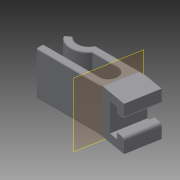
# Autodesk Inventor part: pinza
Saved by Autodesk Inventor 2015 SP1 (Build 190203100, 203)
## iProperties
Created: 2015-12-16
Part Number: pinza
Material: Generic
Document SubType Name: Modeling
Designer: pc
Density: 1 g/cm^3
Appearance: Default
Author: pc
Autodesk Inventor part; units mm, degrees
ref_plane "YZ Plane" through (0, 0, 0) normal (1, 0, 0) x (0, 1, 0)
ref_plane "XZ Plane" through (0, 0, 0) normal (0, 1, 0) x (-1, 0, 0)
ref_plane "XY Plane" through (0, 0, 0) normal (0, 0, 1) x (1, 0, 0)
sketch "Sketch1" plane through (0, 0, 0) normal (0, 0, 1) x (1, 0, 0)
  line L0 (-13.4572, -6) -> (9.0428, -6)
  line L1 (9.0428, -6) -> (9.0428, 0)
  line L2 (9.0428, 0) -> (-2.5, 0)
  arc A0 (-12.5, 0) -> (-2.5, 0) centre (-7.5, 3.75) ccw
  arc A1 (-10.5, 1.5) -> (-3.9645, 2.5) centre (-7.5, 3.75) ccw
  line L3 (-3.9645, 2.5) -> (11.5428, 2.5)
  line L4 (11.5428, 2.5) -> (11.5428, -8.5)
  line L5 (11.5428, -8.5) -> (-13.4572, -8.5)
  line L6 (-13.4572, -6) -> (-13.4572, -8.5)
  line L7 (-12.5, 0) -> (-10.5, 1.5)
  point P0 (0, 0)
  dimension "d4" = 6
  dimension "d5" = 25
  constraints: 16 end point, 4 point on circle, 2 centre point, 2 perpendicular, 1 horizontal, 1 vertical, 3 other
  measures "d4" distance of L0.end L1.end
  measures "d5" distance of L4.end L5.end
extrude "Extrusion1" add sketch "Sketch1" along normal blind 15
ref_plane "Work Plane1" through (11.5428, 2.5, 0) normal (0.9848078, -0.1736482, 0) x (0, 0, 1)
sketch "Sketch3" plane through (0, 0, 0) normal (0, 0, -1) x (-1, 0, 0)
  line L0 (-8.3381, -15.6747) -> (-12.3263, 6.9435) projected
  line L1 (13.4572, -6) -> (-9.0428, -6) projected
  line L2 (-9.0428, -6) -> (-9.0428, 0) projected
  line L3 (-9.0428, 0) -> (2.5, 0) projected
  arc A0 (2.5, 0) -> (12.5, 0) centre (7.5, 3.75) ccw projected
  line L4 (12.5, 0) -> (10.5, 1.5) projected
  arc A1 (3.9645, 2.5) -> (10.5, 1.5) centre (7.5, 3.75) ccw projected
  line L5 (3.9645, 2.5) -> (-11.5428, 2.5) projected
  line L6 (-11.5428, 2.5) -> (-11.5428, -8.5) projected
  line L7 (-11.5428, -8.5) -> (13.4572, -8.5) projected
  line L8 (13.4572, -8.5) -> (13.4572, -6) projected
  line L9 (13.4572, -8.5) -> (-11.5428, -8.5) projected
  line L10 (-9.6032, -8.5) -> (-11.5428, -8.5)
  line L11 (-11.5428, -8.5) -> (-11.5428, 2.5)
  line L12 (-11.5428, 2.5) -> (-9.6032, -8.5)
  point P0 (0, 0)
  constraints: 6 end point, 2 point on line, 1 collinear, 1 perpendicular
extrude "Extrusion2" cut sketch "Sketch3" against normal blind 20 contours L7 L6 L0
sketch "Sketch4" plane through (10.044, -6, 15) normal (0.9848078, -0.1736482, 0) x (0, 0, 1)
  line L0 (0, 2.5386) -> (0, -8.6311) projected
  line L1 (-15, 2.5386) -> (0, 2.5386) projected
  line L2 (-15, -8.6311) -> (-15, 2.5386) projected
  line L3 (-15, -8.6311) -> (-15, 2.5386) projected
  line L4 (-15, -8.6311) -> (0, -8.6311) projected
  line L5 (0, 2.5386) -> (0, -8.6311) projected
  line L6 (-15, 2.5386) -> (-15, -8.6311)
  line L7 (-15, -8.6311) -> (0, -8.6311)
  line L8 (0, -8.6311) -> (0, 2.5386)
  line L9 (-15, 2.5386) -> (0, 2.5386) projected
  line L10 (-15, -8.6311) -> (0, -8.6311) projected
  point P0 (-15, -4.1647)
  constraints: 6 end point, 1 collinear, 1 perpendicular, 1 vertical
extrude "Extrusion3" add sketch "Sketch4" along normal blind 1
sketch "Sketch6" plane through (9.6032, -8.5, 0) normal (-0.1736482, -0.9848078, 0) x (0.9848078, -0.1736482, 0)
  line L0 (1, 15) -> (1, 0) projected
  line L1 (1, 15) -> (9, 15)
  line L2 (9, 15) -> (9, 10.3)
  line L3 (9, 10.3) -> (6, 10.3)
  line L4 (6, 10.3) -> (6, 12.3)
  line L5 (6, 12.3) -> (3, 12.3)
  line L6 (3, 12.3) -> (3, 2.7)
  line L7 (3, 2.7) -> (6, 2.7)
  line L8 (6, 2.7) -> (6, 4.7)
  line L9 (6, 4.7) -> (9, 4.7)
  line L10 (9, 4.7) -> (9, 0)
  line L11 (9, 0) -> (1, 0)
  line L12 (1, 0) -> (1, 15)
  point P0 (-10.9333, 0)
  dimension "d13" = 5.6
  dimension "d14" = 2
  dimension "d15" = 2
  dimension "d16" = 3
  dimension "d17" = 3
  constraints: 24 end point, 9 perpendicular, 4 point on line, 2 collinear, 1 horizontal
  measures "d13" distance of L9.end L2.end
  measures "d14" distance of L3.end L4.end
  measures "d15" distance between parallel lines of L0 L6
  measures "d16" distance of L6.end L7.end
  measures "d17" distance of L8.end L9.end
extrude "Extrusion4" add sketch "Sketch6" against normal up to surface (11.1697 mm away)
fillet "Fillet3" radius 1 2 edges at (19.4363, -4.5628, 4.7) (19.4363, -4.5628, 10.3)
fillet "Fillet1" radius 2.8 2 edges at (9.0428, -6, 7.5) (9.0428, 0, 7.5)
fillet "Fillet2" radius 0.5 28 edges at (-3.6072, -6, 0) (-13.4572, -6, 7.5) (-3.6072, -6, 15) (1.8714, 0, 15) (-2.5, 0, 7.5) (1.8714, 0, 0) (-7.5, -2.5, 0) (-7.5, -2.5, 15) (-12.5, 0, 7.5) (-11.5, 0.75, 0) (-11.5, 0.75, 15) (-10.5, 1.5, 7.5) (-6.9328, 0.0431, 0) (-6.9328, 0.0431, 15) (-3.9645, 2.5, 7.5) (3.7892, 2.5, 0) (3.7892, 2.5, 15) (-1.927, -8.5, 0) (-1.927, -8.5, 15) (-13.4572, -8.5, 7.5) (-13.4572, -7.25, 0) (-13.4572, -7.25, 15) (8.2227, -5.1799, 0) (8.2227, -5.1799, 15) (9.0428, -3, 0) (9.0428, -3, 15) (8.2227, -0.8201, 0) (8.2227, -0.8201, 15)
body "Solid1"
